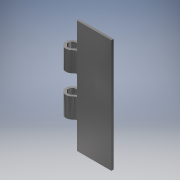
# Autodesk Inventor part: HINGE PLATE 2
Saved by Autodesk Inventor 2017 (Build 210142000, 142)
## iProperties
Created: 2016-08-17
Part Number: HINGE PLATE 2
Material: Stainless Steel
Document SubType Name: Modeling
Designer: Matthewn
Density: 8 g/cm^3
Appearance: Semi-Polished
Author: Matthewn
Autodesk Inventor part; units mm, degrees
ref_plane "YZ Plane" through (0, 0, 0) normal (1, 0, 0) x (0, 1, 0)
ref_plane "XZ Plane" through (0, 0, 0) normal (0, 1, 0) x (-1, 0, 0)
sketch "Sketch1" plane through (0, 0, 0) normal (0, 0, 1) x (1, 0, 0)
  arc A0 (5.6974, 0.1712) -> (4.4165, -3.6034) centre (0, 0) ccw
  line L0 (37.7409, -2.5) -> (6.7409, -2.5)
  arc A1 (3.6983, 0.1111) -> (2.8668, -2.3391) centre (0, 0) ccw
  line L1 (6.7409, -0.5) -> (37.7409, -0.5)
  line L2 (37.7409, -0.5) -> (37.7409, -2.5)
  arc A2 (6.7409, -2.5) -> (4.4165, -3.6034) centre (6.7409, -5.5) ccw
  arc A3 (6.7409, -0.5) -> (2.8668, -2.3391) centre (6.7409, -5.5) ccw
  line L3 (3.6983, 0.1111) -> (5.6974, 0.1712)
  point P0 (5.1225, -2.5)
  dimension "d0" = 11.4
  dimension "d1" = 2
  dimension "d2" = 3
  dimension "d3" = 5
  dimension "d4" = 2
  dimension "d5" = 31
  dimension "d8" = 0.5
  dimension "d9" = 0.7
  constraints: 9 point on circle, 8 end point, 4 centre point, 4 tangent, 2 horizontal, 1 coincident, 1 line through centre, 1 perpendicular, 1 point on line
  measures "d0" diameter of A0
  measures "d1" radial gap between concentric circles of A0 A1
  measures "d2" radius of A2
  measures "d3" radius of A3
  measures "d4" distance between parallel lines of L0 L1
  measures "d5" distance of L0.start L0.end
  measures "d8" distance from line of point (0, 0) L1
  measures "d9" distance edge to line of A3 L3
extrude "Extrusion1" add sketch "Sketch1" along normal mid plane 101.6
ref_plane "Work Plane1" through (0, 0, 27) normal (0, 0, 1) x (1, 0, 0)
sketch "Sketch2" plane through (0, 0, 27) normal (0, 0, 1) x (1, 0, 0)
  arc A0 (6.7409, -2.5) -> (4.4165, -3.6034) centre (6.7409, -5.5) ccw projected
  arc A1 (5.6974, 0.1712) -> (4.4165, -3.6034) centre (0, 0) ccw projected
  line L0 (5.6974, 0.1712) -> (3.6983, 0.1111) projected
  arc A2 (3.6983, 0.1111) -> (2.8668, -2.3391) centre (0, 0) ccw projected
  arc A3 (6.7409, -0.5) -> (2.8668, -2.3391) centre (6.7409, -5.5) ccw projected
  line L1 (6.7409, -0.5) -> (37.7409, -0.5) construction
  line L2 (37.7409, -0.5) -> (37.7409, -2.5) construction
  line L3 (37.7409, -2.5) -> (6.7409, -2.5) construction
  line L4 (6.7409, -0.5) -> (6.7409, -2.5)
  constraints: 2 end point, 1 vertical
extrude "Extrusion2" cut sketch "Sketch2" along normal through all
mirror "Mirror1" about plane through (0, 0, 0) normal (0, 0, 1) of "Extrusion2"
sketch "Sketch3" plane through (0, 0, 0) normal (0, 0, 1) x (1, 0, 0)
  arc A0 (6.7409, -0.5) -> (2.8668, -2.3391) centre (6.7409, -5.5) ccw projected
  line L0 (6.7409, -0.5) -> (37.7409, -0.5) construction
  line L1 (37.7409, -0.5) -> (37.7409, -2.5) projected
  line L2 (37.7409, -2.5) -> (6.7409, -2.5) construction
  arc A1 (6.7409, -2.5) -> (4.4165, -3.6034) centre (6.7409, -5.5) ccw projected
  arc A2 (5.6974, 0.1712) -> (4.4165, -3.6034) centre (0, 0) ccw projected
  line L3 (5.6974, 0.1712) -> (3.6983, 0.1111) projected
  arc A3 (3.6983, 0.1111) -> (2.8668, -2.3391) centre (0, 0) ccw projected
  line L4 (6.7409, -2.5) -> (6.7409, -0.5) projected
  line L5 (6.7409, -2.5) -> (6.7409, -0.5)
  constraints: 2 end point, 1 vertical
extrude "Extrusion3" cut sketch "Sketch3" along normal mid plane 18.1
equation "\"d1\" = d4"
equation "\"d3\" = d2 + d4"
body "Solid1"
